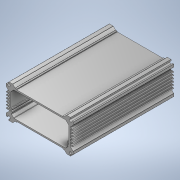
# Autodesk Inventor part: AW11-6-15E
Saved by Autodesk Inventor 2020.2 (Build 242310000, 310)
## iProperties
Created: 2020-06-01
Part Number: AW11-6-15E
Material: Generic
Document SubType Name: Modeling
Designer: ahwv
Density: 1 g/cm^3
Appearance: Anodized - Light Gray
Author: ahwv
Autodesk Inventor part; units mm, degrees
ref_plane "YZ Plane" through (0, 0, 0) normal (1, 0, 0) x (0, 1, 0)
ref_plane "XZ Plane" through (0, 0, 0) normal (0, 1, 0) x (-1, 0, 0)
ref_plane "XY Plane" through (0, 0, 0) normal (0, 0, 1) x (1, 0, 0)
sketch "Sketch1" plane through (0, 0, 0) normal (0, 0, 1) x (1, 0, 0)
  line L0 (-44.428, -19.8994) -> (-39.428, -19.8994)
  line L1 (-44.428, 22.3006) -> (-44.428, 27.3006)
  line L2 (47.772, 22.3006) -> (52.772, 22.3006)
  line L3 (47.772, 22.3006) -> (47.772, 27.3006)
  line L4 (47.772, 22.3006) -> (47.772, 17.3006)
  line L5 (47.772, -19.8994) -> (47.772, -24.8994)
  line L6 (47.772, 22.3006) -> (42.772, 22.3006)
  line L7 (-44.428, 22.3006) -> (-39.428, 22.3006)
  line L8 (47.772, -19.8994) -> (42.772, -19.8994)
  line L9 (47.772, -19.8994) -> (47.772, -14.8994)
  line L10 (-44.428, 22.3006) -> (-44.428, 17.3006)
  line L11 (47.772, -19.8994) -> (52.772, -19.8994)
  line L12 (-44.428, -19.8994) -> (-44.428, -14.8994)
  line L13 (-44.428, 22.3006) -> (-49.428, 22.3006)
  line L14 (-44.428, -19.8994) -> (-44.428, -24.8994)
  line L15 (-44.428, -19.8994) -> (-49.428, -19.8994)
  arc A0 (47.672, -10.2994) -> (47.172, -10.7994) centre (47.672, -10.7994) ccw
  line L16 (47.172, -11.0923) -> (47.172, -10.7994)
  arc A1 (47.172, -11.0923) -> (47.3185, -11.4458) centre (47.672, -11.0923) ccw
  line L17 (51.5256, -15.6529) -> (47.3185, -11.4458)
  arc A2 (51.672, -16.0065) -> (51.5256, -15.6529) centre (51.172, -16.0065) ccw
  line L18 (51.672, -19.6904) -> (51.672, -16.0065)
  arc A3 (49.4535, -19.649) -> (49.5006, -19.8441) centre (50.5662, -19.4834) ccw
  arc A4 (49.5006, -19.8441) -> (51.672, -19.6904) centre (50.5662, -19.4834) ccw
  arc A5 (49.4535, -19.649) -> (47.5217, -21.5808) centre (47.772, -19.8994) ccw
  arc A6 (49.5006, -19.8441) -> (47.7168, -21.628) centre (47.772, -19.8994) ccw
  arc A7 (47.563, -23.7994) -> (47.7168, -21.628) centre (47.356, -22.6936) ccw
  arc A8 (47.7168, -21.628) -> (47.5217, -21.5808) centre (47.356, -22.6936) ccw
  line L19 (47.672, -6.0494) -> (50.797, -6.0494)
  line L20 (50.797, -4.2994) -> (47.672, -4.2994)
  arc A9 (50.797, -6.0494) -> (50.797, -4.2994) centre (50.797, -5.1744) ccw
  arc A10 (47.172, -3.7994) -> (47.672, -4.2994) centre (47.672, -3.7994) ccw
  line L21 (47.172, -3.7994) -> (47.172, -2.2994)
  line L22 (47.672, -1.7994) -> (50.797, -1.7994)
  arc A11 (47.672, -1.7994) -> (47.172, -2.2994) centre (47.672, -2.2994) ccw
  arc A12 (47.672, -6.0494) -> (47.172, -6.5494) centre (47.672, -6.5494) ccw
  arc A13 (40.7149, 19.1577) -> (40.0078, 19.4506) centre (40.0078, 18.4506) ccw
  arc A14 (40.0078, -17.0494) -> (40.7149, -16.7565) centre (40.0078, -16.0494) ccw
  line L23 (41.7755, 26.0542) -> (38.5098, 22.7885)
  arc A15 (38.2977, 22.7006) -> (38.5098, 22.7885) centre (38.2977, 23.0006) ccw
  line L24 (38.2977, 22.7006) -> (36.222, 22.7006)
  line L25 (35.922, -19.2994) -> (35.922, -19.9994)
  line L26 (36.222, -20.2994) -> (38.2977, -20.2994)
  line L27 (35.922, 21.7006) -> (-32.578, 21.7006)
  arc A16 (-32.578, 22.4006) -> (-32.878, 22.7006) centre (-32.878, 22.4006) ccw
  line L28 (-36.6638, 19.4506) -> (40.0078, 19.4506)
  arc A17 (-38.4314, 26.0542) -> (-38.785, 26.2006) centre (-38.785, 25.7006) ccw
  line L29 (-48.1815, 18.0542) -> (-43.9744, 13.8471)
  arc A18 (-43.828, 13.4935) -> (-43.9744, 13.8471) centre (-44.328, 13.4935) ccw
  line L30 (40.0078, -17.0494) -> (-36.6638, -17.0494)
  line L31 (-32.578, -19.2994) -> (35.922, -19.2994)
  arc A19 (-32.878, -20.2994) -> (-32.578, -19.9994) centre (-32.878, -19.9994) ccw
  arc A20 (35.922, -19.9994) -> (36.222, -20.2994) centre (36.222, -19.9994) ccw
  arc A21 (44.922, 14.5364) -> (44.6291, 15.2435) centre (43.922, 14.5364) ccw
  arc A22 (43.6291, -13.8423) -> (43.922, -13.1351) centre (42.922, -13.1351) ccw
  line L32 (43.6291, -13.8423) -> (40.7149, -16.7565)
  arc A23 (47.172, 4.7006) -> (47.672, 4.2006) centre (47.672, 4.7006) ccw
  arc A24 (47.172, 13.2006) -> (47.672, 12.7006) centre (47.672, 13.2006) ccw
  line L33 (47.672, 10.9506) -> (50.797, 10.9506)
  line L34 (47.3185, 13.8471) -> (51.5256, 18.0542)
  arc A25 (50.797, 6.7006) -> (50.797, 8.4506) centre (50.797, 7.5756) ccw
  arc A26 (51.5256, 18.0542) -> (51.672, 18.4077) centre (51.172, 18.4077) ccw
  arc A27 (47.3185, 13.8471) -> (47.172, 13.4935) centre (47.672, 13.4935) ccw
  line L35 (47.172, 13.2006) -> (47.172, 13.4935)
  arc A28 (47.672, 10.9506) -> (47.172, 10.4506) centre (47.672, 10.4506) ccw
  line L36 (47.172, 8.9506) -> (47.172, 10.4506)
  arc A29 (47.172, 8.9506) -> (47.672, 8.4506) centre (47.672, 8.9506) ccw
  line L37 (47.563, 26.2006) -> (42.129, 26.2006)
  arc A30 (42.129, 26.2006) -> (41.7755, 26.0542) centre (42.129, 25.7006) ccw
  arc A31 (47.672, 6.7006) -> (47.172, 6.2006) centre (47.672, 6.2006) ccw
  arc A32 (49.5006, 22.2454) -> (49.4535, 22.0503) centre (50.5662, 21.8847) ccw
  arc A33 (51.672, 22.0916) -> (49.5006, 22.2454) centre (50.5662, 21.8847) ccw
  arc A34 (47.5217, 23.9821) -> (47.7168, 24.0293) centre (47.356, 25.0948) ccw
  arc A35 (47.5217, 23.9821) -> (49.4535, 22.0503) centre (47.772, 22.3006) ccw
  arc A36 (47.7168, 24.0293) -> (47.563, 26.2006) centre (47.356, 25.0948) ccw
  arc A37 (47.7168, 24.0293) -> (49.5006, 22.2454) centre (47.772, 22.3006) ccw
  line L38 (35.922, 22.4006) -> (35.922, 21.7006)
  arc A38 (36.222, 22.7006) -> (35.922, 22.4006) centre (36.222, 22.4006) ccw
  arc A39 (-48.328, 18.4077) -> (-48.1815, 18.0542) centre (-47.828, 18.4077) ccw
  line L39 (42.922, -6.8494) -> (42.922, -7.5994)
  line L40 (42.922, -10.6994) -> (42.922, -11.4494)
  line L41 (40.7149, 19.1577) -> (44.6291, 15.2435)
  arc A40 (43.422, -10.1994) -> (42.922, -10.6994) centre (43.422, -10.6994) ccw
  arc A41 (42.922, -11.4494) -> (43.422, -11.9494) centre (43.422, -11.4494) ccw
  line L42 (43.922, -12.4494) -> (43.922, -13.1351)
  arc A42 (43.922, -12.4494) -> (43.422, -11.9494) centre (43.422, -12.4494) ccw
  arc A43 (43.422, -6.3494) -> (42.922, -6.8494) centre (43.422, -6.8494) ccw
  arc A44 (42.922, -7.5994) -> (43.422, -8.0994) centre (43.422, -7.5994) ccw
  line L43 (44.422, -6.3494) -> (43.422, -6.3494)
  line L44 (44.922, -10.0494) -> (43.422, -10.1994)
  line L45 (44.922, -8.2494) -> (44.922, -10.0494)
  line L46 (43.422, -8.0994) -> (44.922, -8.2494)
  arc A45 (44.422, -6.3494) -> (44.922, -5.8494) centre (44.422, -5.8494) ccw
  line L47 (44.922, 14.5364) -> (44.922, -5.8494)
  line L48 (47.172, 4.7006) -> (47.172, 6.2006)
  line L49 (47.172, 0.4506) -> (47.172, 1.9506)
  arc A46 (47.672, 2.4506) -> (47.172, 1.9506) centre (47.672, 1.9506) ccw
  arc A47 (47.172, 0.4506) -> (47.672, -0.0494) centre (47.672, 0.4506) ccw
  line L50 (51.672, 18.4077) -> (51.672, 22.0916)
  line L51 (50.797, 4.2006) -> (47.672, 4.2006)
  line L52 (47.672, 2.4506) -> (50.797, 2.4506)
  line L53 (47.672, 6.7006) -> (50.797, 6.7006)
  line L54 (50.797, 8.4506) -> (47.672, 8.4506)
  line L55 (50.797, -0.0494) -> (47.672, -0.0494)
  arc A48 (50.797, -1.7994) -> (50.797, -0.0494) centre (50.797, -0.9244) ccw
  arc A49 (50.797, 2.4506) -> (50.797, 4.2006) centre (50.797, 3.3256) ccw
  arc A50 (50.797, 10.9506) -> (50.797, 12.7006) centre (50.797, 11.8256) ccw
  line L56 (50.797, 12.7006) -> (47.672, 12.7006)
  line L57 (47.172, -8.0494) -> (47.172, -6.5494)
  arc A51 (47.172, -8.0494) -> (47.672, -8.5494) centre (47.672, -8.0494) ccw
  line L58 (50.797, -8.5494) -> (47.672, -8.5494)
  arc A52 (50.797, -10.2994) -> (50.797, -8.5494) centre (50.797, -9.4244) ccw
  line L59 (47.672, -10.2994) -> (50.797, -10.2994)
  line L60 (42.129, -23.7994) -> (47.563, -23.7994)
  arc A53 (41.7755, -23.6529) -> (42.129, -23.7994) centre (42.129, -23.2994) ccw
  line L61 (38.5098, -20.3872) -> (41.7755, -23.6529)
  arc A54 (38.5098, -20.3872) -> (38.2977, -20.2994) centre (38.2977, -20.5994) ccw
  arc A55 (-37.3709, -16.7565) -> (-36.6638, -17.0494) centre (-36.6638, -16.0494) ccw
  line L62 (-37.3709, -16.7565) -> (-40.2851, -13.8423)
  arc A56 (-40.578, -13.1351) -> (-40.2851, -13.8423) centre (-39.578, -13.1351) ccw
  arc A57 (-41.2851, 15.2435) -> (-41.578, 14.5364) centre (-40.578, 14.5364) ccw
  line L63 (-41.578, -5.8494) -> (-41.578, 14.5364)
  line L64 (-44.328, -0.0494) -> (-47.453, -0.0494)
  arc A58 (-44.328, -0.0494) -> (-43.828, 0.4506) centre (-44.328, 0.4506) ccw
  line L65 (-43.828, 1.9506) -> (-43.828, 0.4506)
  arc A59 (-43.828, 1.9506) -> (-44.328, 2.4506) centre (-44.328, 1.9506) ccw
  line L66 (-47.453, 2.4506) -> (-44.328, 2.4506)
  line L67 (-44.328, 4.2006) -> (-47.453, 4.2006)
  arc A60 (-44.328, 4.2006) -> (-43.828, 4.7006) centre (-44.328, 4.7006) ccw
  line L68 (-43.828, 6.2006) -> (-43.828, 4.7006)
  arc A61 (-43.828, 6.2006) -> (-44.328, 6.7006) centre (-44.328, 6.2006) ccw
  line L69 (-44.328, 8.4506) -> (-47.453, 8.4506)
  arc A62 (-44.328, 8.4506) -> (-43.828, 8.9506) centre (-44.328, 8.9506) ccw
  line L70 (-43.828, 10.4506) -> (-43.828, 8.9506)
  arc A63 (-43.828, 10.4506) -> (-44.328, 10.9506) centre (-44.328, 10.4506) ccw
  line L71 (-47.453, 10.9506) -> (-44.328, 10.9506)
  line L72 (-44.328, 12.7006) -> (-47.453, 12.7006)
  arc A64 (-44.328, 12.7006) -> (-43.828, 13.2006) centre (-44.328, 13.2006) ccw
  line L73 (-43.828, 13.4935) -> (-43.828, 13.2006)
  line L74 (-47.453, 6.7006) -> (-44.328, 6.7006)
  arc A65 (-41.578, -5.8494) -> (-41.078, -6.3494) centre (-41.078, -5.8494) ccw
  line L75 (-40.078, -6.3494) -> (-41.078, -6.3494)
  arc A66 (-39.578, -6.8494) -> (-40.078, -6.3494) centre (-40.078, -6.8494) ccw
  line L76 (-39.578, -7.5994) -> (-39.578, -6.8494)
  arc A67 (-40.078, -8.0994) -> (-39.578, -7.5994) centre (-40.078, -7.5994) ccw
  line L77 (-41.578, -8.2494) -> (-40.078, -8.0994)
  line L78 (-47.453, -1.7994) -> (-44.328, -1.7994)
  arc A68 (-43.828, -2.2994) -> (-44.328, -1.7994) centre (-44.328, -2.2994) ccw
  line L79 (-43.828, -2.2994) -> (-43.828, -3.7994)
  arc A69 (-44.328, -4.2994) -> (-43.828, -3.7994) centre (-44.328, -3.7994) ccw
  line L80 (-44.328, -4.2994) -> (-47.453, -4.2994)
  line L81 (-47.453, -6.0494) -> (-44.328, -6.0494)
  arc A70 (-43.828, -6.5494) -> (-44.328, -6.0494) centre (-44.328, -6.5494) ccw
  line L82 (-43.828, -6.5494) -> (-43.828, -8.0494)
  line L83 (-44.328, -8.5494) -> (-47.453, -8.5494)
  line L84 (-47.453, -10.2994) -> (-44.328, -10.2994)
  line L85 (-41.578, -10.0494) -> (-41.578, -8.2494)
  arc A71 (-43.828, -10.7994) -> (-44.328, -10.2994) centre (-44.328, -10.7994) ccw
  line L86 (-43.828, -10.7994) -> (-43.828, -11.0923)
  arc A72 (-43.9744, -11.4458) -> (-43.828, -11.0923) centre (-44.328, -11.0923) ccw
  arc A73 (-44.328, -8.5494) -> (-43.828, -8.0494) centre (-44.328, -8.0494) ccw
  arc A74 (-44.3728, 24.0293) -> (-44.1776, 23.9821) centre (-44.012, 25.0948) ccw
  arc A75 (-46.1094, 22.0503) -> (-44.1776, 23.9821) centre (-44.428, 22.3006) ccw
  arc A76 (-46.1566, 22.2454) -> (-44.3728, 24.0293) centre (-44.428, 22.3006) ccw
  arc A77 (-44.219, 26.2006) -> (-44.3728, 24.0293) centre (-44.012, 25.0948) ccw
  arc A78 (-46.1094, 22.0503) -> (-46.1566, 22.2454) centre (-47.2222, 21.8847) ccw
  line L87 (-32.578, 21.7006) -> (-32.578, 22.4006)
  line L88 (-32.878, 22.7006) -> (-34.9536, 22.7006)
  line L89 (-35.1657, 22.7885) -> (-38.4314, 26.0542)
  line L90 (-38.785, 26.2006) -> (-44.219, 26.2006)
  line L91 (-48.328, 22.0916) -> (-48.328, 18.4077)
  line L92 (-40.078, -10.1994) -> (-41.578, -10.0494)
  arc A79 (-39.578, -10.6994) -> (-40.078, -10.1994) centre (-40.078, -10.6994) ccw
  line L93 (-39.578, -11.4494) -> (-39.578, -10.6994)
  arc A80 (-40.078, -11.9494) -> (-39.578, -11.4494) centre (-40.078, -11.4494) ccw
  arc A81 (-40.078, -11.9494) -> (-40.578, -12.4494) centre (-40.078, -12.4494) ccw
  line L94 (-40.578, -13.1351) -> (-40.578, -12.4494)
  line L95 (-32.578, -19.9994) -> (-32.578, -19.2994)
  line L96 (-34.9536, -20.2994) -> (-32.878, -20.2994)
  arc A82 (-34.9536, -20.2994) -> (-35.1657, -20.3872) centre (-34.9536, -20.5994) ccw
  line L97 (-38.4314, -23.6529) -> (-35.1657, -20.3872)
  arc A83 (-38.785, -23.7994) -> (-38.4314, -23.6529) centre (-38.785, -23.2994) ccw
  line L98 (-44.219, -23.7994) -> (-38.785, -23.7994)
  line L99 (-43.9744, -11.4458) -> (-48.1815, -15.6529)
  arc A84 (-44.1776, -21.5808) -> (-46.1094, -19.649) centre (-44.428, -19.8994) ccw
  arc A85 (-44.1776, -21.5808) -> (-44.3728, -21.628) centre (-44.012, -22.6936) ccw
  arc A86 (-44.3728, -21.628) -> (-44.219, -23.7994) centre (-44.012, -22.6936) ccw
  arc A87 (-44.3728, -21.628) -> (-46.1566, -19.8441) centre (-44.428, -19.8994) ccw
  line L100 (-48.328, -16.0065) -> (-48.328, -19.6904)
  arc A88 (-48.1815, -15.6529) -> (-48.328, -16.0065) centre (-47.828, -16.0065) ccw
  arc A89 (-47.453, -8.5494) -> (-47.453, -10.2994) centre (-47.453, -9.4244) ccw
  arc A90 (-47.453, -4.2994) -> (-47.453, -6.0494) centre (-47.453, -5.1744) ccw
  arc A91 (-47.453, -0.0494) -> (-47.453, -1.7994) centre (-47.453, -0.9244) ccw
  arc A92 (-47.453, 4.2006) -> (-47.453, 2.4506) centre (-47.453, 3.3256) ccw
  arc A93 (-47.453, 8.4506) -> (-47.453, 6.7006) centre (-47.453, 7.5756) ccw
  arc A94 (-47.453, 12.7006) -> (-47.453, 10.9506) centre (-47.453, 11.8256) ccw
  arc A95 (-48.328, -19.6904) -> (-46.1566, -19.8441) centre (-47.2222, -19.4834) ccw
  arc A96 (-46.1566, 22.2454) -> (-48.328, 22.0916) centre (-47.2222, 21.8847) ccw
  arc A97 (-46.1566, -19.8441) -> (-46.1094, -19.649) centre (-47.2222, -19.4834) ccw
  arc A98 (-36.6638, 19.4506) -> (-37.3709, 19.1577) centre (-36.6638, 18.4506) ccw
  line L101 (-41.2851, 15.2435) -> (-37.3709, 19.1577)
  arc A99 (-35.1657, 22.7885) -> (-34.9536, 22.7006) centre (-34.9536, 23.0006) ccw
  arc A100 (49.7413, -20.2484) -> (48.121, -21.8687) centre (47.772, -19.8994) ccw
  arc A101 (-46.3973, 22.6496) -> (-44.777, 24.27) centre (-44.428, 22.3006) ccw
  arc A102 (48.121, 24.27) -> (49.7413, 22.6496) centre (47.772, 22.3006) ccw
  arc A103 (-44.777, -21.8687) -> (-46.3973, -20.2484) centre (-44.428, -19.8994) ccw
  point P0 (0, 0)
  point P1 (51.6115, 22.3006)
  point P2 (49.772, 22.3006)
  point P3 (47.772, 24.3006)
  point P4 (47.772, 26.1401)
  point P5 (-44.428, 26.1401)
  point P6 (-44.428, 24.3006)
  point P7 (-46.428, 22.3006)
  point P8 (-48.2674, 22.3006)
  point P9 (-48.2674, -19.8994)
  point P10 (-46.428, -19.8994)
  point P11 (-44.428, -21.8994)
  point P12 (-44.428, -23.7388)
  point P13 (47.772, -23.7388)
  point P14 (47.772, -21.8994)
  point P15 (49.772, -19.8994)
  point P16 (51.6115, -19.8994)
  dimension "d1" = 36.5
  dimension "d3" = 86.5
  dimension "d5" = 7
  dimension "d7" = 1.8
  dimension "d8" = 41
  dimension "d9" = 100
  dimension "d10" = 91
  dimension "d11" = 2.25
  constraints: 216 point on circle, 204 end point, 104 centre point
  measures "d1" distance between parallel lines of L28 L30
  measures "d3" distance between parallel lines of L63 L47
  measures "d5" vertical distance of L30.end L85.start
  measures "d7" distance of L85.start L77.start
  measures "d8" distance between parallel lines of L31 L27
  measures "d9" distance between parallel lines of L18 L100
  measures "d10" distance between parallel lines of L36 L70
  measures "d11" distance between parallel lines of L31 L30
extrude "Extrusion1" add sketch "Sketch1" along normal blind 150 contours A103 L15 A95 L100 A88 L99 A72 L86 A71 L84 A89 L83 A73 L82 A70 L81 A90 L80 A69 L79 A68 L78 A91 L64 A58 L65 A59 L66 A92 L67 A60 L68 A61 L74 A93 L69 A62 L70 A63 L71 A94 L72 A64 L73 A18 L29 A39 L91 A96 L13 A101 L1 A77 L90 A17 L89 A99 L88 A16 L87 L27 L38 A38 L24 A15 L23 A30 L37 A36 L3 A102 L2 A33 L50 A26 L34 A27 L35 A24 L56 A50 L33 A28 L36 A29 L54 A25 L53 A31 L48 A23 L51 A49 L52 A46 L49 A47 L55 A48 L22 A11 L21 A10 L20 A9 L19 A12 L57 A51 L58 A52 L59 A0 L16 A1 L17 A2 L18 A4 L11 A100 L5 A7 L60 A53 L61 A54 L26 A20 L25 L31 L95 A19 L96 A82 L97 A83 L98 A86 L14
body "Solid1"
